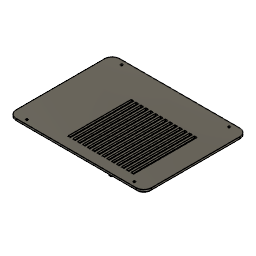
Mini PC Lid V2 (Autodesk Fusion 360 design; units mm, degrees)
Autodesk Fusion 360 part; units mm, degrees
sketch "Sketch1" plane through (0, 0, 0) normal (0, 0, 1) x (1, 0, 0)
  line L0 (10, 0) -> (200, 0)
  line L1 (210, 10) -> (210, 150)
  line L2 (200, 160) -> (10, 160)
  line L3 (0, 150) -> (0, 10)
  arc A0 (10, 160) -> (0, 150) centre (10, 150) ccw
  arc A1 (210, 150) -> (200, 160) centre (200, 150) ccw
  arc A2 (200, 0) -> (210, 10) centre (200, 10) ccw
  arc A3 (0, 10) -> (10, 0) centre (10, 10) ccw
  line L4 (200, 162) -> (10, 162)
  arc A4 (10, 162) -> (-2, 150) centre (10, 150) ccw
  line L5 (-2, 150) -> (-2, 10)
  arc A5 (-2, 10) -> (10, -2) centre (10, 10) ccw
  line L6 (10, -2) -> (200, -2)
  arc A6 (200, -2) -> (212, 10) centre (200, 10) ccw
  line L7 (212, 10) -> (212, 150)
  arc A7 (212, 150) -> (200, 162) centre (200, 150) ccw
  line L8 (200, 155) -> (10, 155)
  arc A8 (10, 155) -> (5, 150) centre (10, 150) ccw
  line L9 (5, 150) -> (5, 10)
  arc A9 (5, 10) -> (10, 5) centre (10, 10) ccw
  line L10 (10, 5) -> (200, 5)
  arc A10 (200, 5) -> (205, 10) centre (200, 10) ccw
  line L11 (205, 10) -> (205, 150)
  arc A11 (205, 150) -> (200, 155) centre (200, 150) ccw
  circle A12 centre (20, 5) radius 1.1
  circle A13 centre (20, 5) radius 3
  circle A14 centre (66, 85) radius 1.1
  circle A15 centre (186, 76) radius 1.1
  circle A16 centre (150, 9) radius 1.1
  circle A17 centre (150, 9) radius 3
  circle A18 centre (66, 85) radius 3
  circle A19 centre (186, 76) radius 3
  line L12 (105, 162) -> (105, -2) construction
  line L13 (212, 80) -> (-2, 80) construction
  circle A20 centre (190, 5) radius 3
  circle A21 centre (190, 5) radius 1.1
  circle A22 centre (20, 155) radius 3
  circle A23 centre (20, 155) radius 1.1
  circle A24 centre (190, 155) radius 3
  circle A25 centre (190, 155) radius 1.1
  point P0 (210, 0)
  point P1 (0, 160)
  dimension "d1" = 210
  dimension "d2" = 160
  dimension "d4" = 10
  dimension "d5" = 2
  dimension "d6" = -5
  dimension "d9" = 2.2
  dimension "d10" = 6
  dimension "d11" = 20
  dimension "d12" = 5
  dimension "d13" = 2.2
  dimension "d14" = 2.2
  dimension "d15" = 2.2
  dimension "d17" = 75
  dimension "d18" = 84
  dimension "d19" = 24
  dimension "d21" = 60
  dimension "d22" = 9
  dimension "d23" = 66
  dimension "d24" = 6
  dimension "d25" = 6
  dimension "d26" = 6
  dimension "d31" = 170
  dimension "d32" = 150
  constraint horizontal L0
  constraint vertical L1
  constraint horizontal L2
  constraint vertical L3
  constraint coincident P1 L2
  constraint coincident P1 L3
  constraint tangent L2 A0
  constraint tangent L3 A0
  constraint tangent L1 A1
  constraint tangent L2 A1
  constraint equal A0 A1
  constraint coincident P0 L0
  constraint coincident P0 L1
  constraint tangent L0 A2
  constraint tangent L1 A2
  constraint equal A0 A2
  constraint coincident origin L0
  constraint coincident origin L3
  constraint tangent L0 A3
  constraint tangent L3 A3
  constraint equal A0 A3
  constraint concentric A12 A13
  constraint concentric A16 A17
  constraint concentric A14 A18
  constraint concentric A15 A19
  constraint midpoint L4 L12.start
  constraint midpoint L6 L12.end
  constraint midpoint L7 L13.start
  constraint midpoint L5 L13.end
  measures "d1" distance of origin P0
  measures "d2" distance of origin P1
  measures "d4" radius of A0
  measures "d9" diameter of A12
  measures "d10" diameter of A13
  measures "d11" distance of L3 A12.centre
  measures "d12" distance of L0 A12.centre
  measures "d13" diameter of A14
  measures "d14" diameter of A15
  measures "d15" diameter of A16
  measures "d17" distance of L2 A14.centre
  measures "d18" distance of L2 A15.centre
  measures "d19" distance of L1 A15.centre
  measures "d21" distance of L1 A16.centre
  measures "d22" distance of L0 A16.centre
  measures "d23" distance of L3 A14.centre
  measures "d24" diameter of A17
  measures "d25" diameter of A18
  measures "d26" diameter of A19
extrude "Extrude1" add sketch "Sketch1" against normal blind 1 contours L0 L1 L2 L3 A0 A1 A2 A3 | L4 A4 L5 A5 L6 A6 L7 A7 | L8 A8 L9 A9 L10 A10 L11 A11 A13 A20 A22 A24 | L8 A24 A25 | L8 A24 A25 | L8 A25 | L8 A25 | L8 A22 A23 | L8 A22 A23 | L8 A23 | L8 A23 | L10 A20 A21 | L10 A20 A21 | L10 A21 | L10 A21 | L10 A12 A13 | L10 A12 A13 | L10 A12 | L10 A12 | A14 | A15 | A16 | A17 | A18 | A19
extrude "Extrude2" add sketch "Sketch1" against normal blind 3 contours L0 L1 L2 L3 A0 A1 A2 A3 | L8 A24 A25 | L8 A24 A25 | L8 A22 A23 | L8 A22 A23 | L10 A20 A21 | L10 A20 A21 | L10 A12 A13 | L10 A12 A13 | A17 | A18 | A19
sketch "Sketch3" plane through (0, 0, -1) normal (0, 0, -1) x (1, 0, 0)
  arc A0 (200, -162) -> (212, -150) centre (200, -150) ccw
  line L0 (212, -150) -> (212, -10)
  arc A1 (212, -10) -> (200, 2) centre (200, -10) ccw
  line L1 (200, 2) -> (10, 2)
  arc A2 (10, 2) -> (-2, -10) centre (10, -10) ccw
  line L2 (-2, -10) -> (-2, -150)
  arc A3 (-2, -150) -> (10, -162) centre (10, -150) ccw
  line L3 (10, -162) -> (200, -162)
  circle A4 centre (190, -155) radius 2.25
  circle A5 centre (20, -155) radius 2.25
  circle A6 centre (66, -85) radius 2.25
  circle A7 centre (186, -76) radius 2.25
  circle A8 centre (190, -5) radius 2.25
  circle A9 centre (150, -9) radius 2.25
  circle A10 centre (20, -5) radius 2.25
  line L4 (10, 0) -> (200, 0)
  arc A11 (210, -10) -> (200, 0) centre (200, -10) ccw
  line L5 (210, -10) -> (210, -150)
  arc A12 (200, -160) -> (210, -150) centre (200, -150) ccw
  line L6 (200, -160) -> (10, -160)
  arc A13 (0, -150) -> (10, -160) centre (10, -150) ccw
  line L7 (0, -150) -> (0, -10)
  arc A14 (10, 0) -> (0, -10) centre (10, -10) ccw
  dimension "d38" = 4.5
  dimension "d39" = 4.5
  dimension "d40" = 4.5
  dimension "d41" = 4.5
  dimension "d42" = 4.5
  dimension "d43" = 4.5
  dimension "d44" = 4.5
  measures "d38" diameter of A4
  measures "d39" diameter of A5
  measures "d40" diameter of A6
  measures "d41" diameter of A7
  measures "d42" diameter of A8
  measures "d43" diameter of A9
  measures "d44" diameter of A10
extrude "Extrude5" cut 4 faces at (189.4633, 4.7506, -1) (20.2286, 5.396, -1) (20.2286, 154.7133, -1) (189.8112, 154.6587, -1) along direction (0, 0, -1) up to surface end surface through (0, 0, 0) normal (0, 0, 1) offset 0
chamfer "Chamfer1" distance 0.5 angle 45 4 edges at (188.9744, 155.3978, 0) (188.9744, 5.3978, 0) (18.9744, 5.3978, 0) (18.9744, 155.3978, 0)
extrude "Extrude6" add 3 faces at (184.3747, 74.2886, -3) (152.3555, 8.851, -3) (64.3747, 83.2886, -3) along direction (0, 0, -1) blind 8
chamfer "Chamfer2" distance 2 angle 45 3 edges at (183.203, 74.9152, -1) (147.203, 7.9152, -1) (63.203, 83.9152, -1)
sketch "Sketch4" plane through (0, 0, -1) normal (0, 0, -1) x (1, 0, 0)
  circle A0 centre (186, -76) radius 5
  arc A1 (147, -5) -> (153, -5) centre (150, -9) ccw
  line L0 (147, -5) -> (23, -5)
  arc A2 (17, -5) -> (23, -5) centre (20, -5) ccw
  line L1 (17, -5) -> (10, -5)
  arc A3 (10, -5) -> (5, -10) centre (10, -10) ccw
  line L2 (5, -10) -> (5, -150)
  arc A4 (5, -150) -> (10, -155) centre (10, -150) ccw
  line L3 (10, -155) -> (17, -155)
  arc A5 (23, -155) -> (17, -155) centre (20, -155) ccw
  line L4 (23, -155) -> (187, -155)
  arc A6 (193, -155) -> (187, -155) centre (190, -155) ccw
  line L5 (193, -155) -> (200, -155)
  arc A7 (200, -155) -> (205, -150) centre (200, -150) ccw
  line L6 (205, -150) -> (205, -10)
  arc A8 (205, -10) -> (200, -5) centre (200, -10) ccw
  line L7 (200, -5) -> (193, -5)
  arc A9 (187, -5) -> (193, -5) centre (190, -5) ccw
  line L8 (187, -5) -> (153, -5)
  circle A10 centre (66, -85) radius 5
  line L9 (75, -115) -> (79, -115)
  line L10 (79, -115) -> (79, -15)
  line L11 (79, -15) -> (75, -15)
  line L12 (75, -15) -> (75, -115)
  line L13 (82.6923, -15) -> (82.6923, -115)
  line L14 (82.6923, -115) -> (86.6923, -115)
  line L15 (86.6923, -115) -> (86.6923, -15)
  line L16 (86.6923, -15) -> (82.6923, -15)
  line L17 (90.3846, -15) -> (90.3846, -115)
  line L18 (90.3846, -115) -> (94.3846, -115)
  line L19 (94.3846, -115) -> (94.3846, -15)
  line L20 (94.3846, -15) -> (90.3846, -15)
  line L21 (98.0769, -15) -> (98.0769, -115)
  line L22 (98.0769, -115) -> (102.0769, -115)
  line L23 (102.0769, -115) -> (102.0769, -15)
  line L24 (102.0769, -15) -> (98.0769, -15)
  line L25 (105.7692, -15) -> (105.7692, -115)
  line L26 (105.7692, -115) -> (109.7692, -115)
  line L27 (109.7692, -115) -> (109.7692, -15)
  line L28 (109.7692, -15) -> (105.7692, -15)
  line L29 (113.4615, -15) -> (113.4615, -115)
  line L30 (113.4615, -115) -> (117.4615, -115)
  line L31 (117.4615, -115) -> (117.4615, -15)
  line L32 (117.4615, -15) -> (113.4615, -15)
  line L33 (121.1538, -15) -> (121.1538, -115)
  line L34 (121.1538, -115) -> (125.1538, -115)
  line L35 (125.1538, -115) -> (125.1538, -15)
  line L36 (125.1538, -15) -> (121.1538, -15)
  line L37 (128.8462, -15) -> (128.8462, -115)
  line L38 (128.8462, -115) -> (132.8462, -115)
  line L39 (132.8462, -115) -> (132.8462, -15)
  line L40 (132.8462, -15) -> (128.8462, -15)
  line L41 (136.5385, -15) -> (136.5385, -115)
  line L42 (136.5385, -115) -> (140.5385, -115)
  line L43 (140.5385, -115) -> (140.5385, -15)
  line L44 (140.5385, -15) -> (136.5385, -15)
  line L45 (144.2308, -15) -> (144.2308, -115)
  line L46 (144.2308, -115) -> (148.2308, -115)
  line L47 (148.2308, -115) -> (148.2308, -15)
  line L48 (148.2308, -15) -> (144.2308, -15)
  line L49 (151.9231, -15) -> (151.9231, -115)
  line L50 (151.9231, -115) -> (155.9231, -115)
  line L51 (155.9231, -115) -> (155.9231, -15)
  line L52 (155.9231, -15) -> (151.9231, -15)
  line L53 (159.6154, -15) -> (159.6154, -115)
  line L54 (159.6154, -115) -> (163.6154, -115)
  line L55 (163.6154, -115) -> (163.6154, -15)
  line L56 (163.6154, -15) -> (159.6154, -15)
  line L57 (167.3077, -15) -> (167.3077, -115)
  line L58 (167.3077, -115) -> (171.3077, -115)
  line L59 (171.3077, -115) -> (171.3077, -15)
  line L60 (171.3077, -15) -> (167.3077, -15)
  line L61 (175, -15) -> (175, -115)
  line L62 (175, -115) -> (179, -115)
  line L63 (179, -115) -> (179, -15)
  line L64 (179, -15) -> (175, -15)
  dimension "d53" = 4
  dimension "d54" = 100
  dimension "d57" = 100
  dimension "d58" = 0
  constraint horizontal L9
  constraint vertical L10
  constraint horizontal L11
  constraint vertical L12
  measures "d53" distance of L9.start L9.end
  measures "d54" distance of L9.start L11.end
extrude "Extrude7" cut sketch "Sketch4" against normal blind 2 contours L9 L10 L11 L12 | L13 L14 L15 L16 | L17 L18 L19 L20 | L21 L22 L23 L24 | L25 L26 L27 L28 | L29 L30 L31 L32 | L33 L34 L35 L36 | L37 L38 L39 L40 | L41 L42 L43 L44 | L45 L46 L47 L48 | L49 L50 L51 L52 | L53 L54 L55 L56 | L57 L58 L59 L60 | L61 L62 L63 L64
extrude "Extrude8" add 1 faces at (23.6667, 91.6667, 0) along direction (0, 0, 1) blind 2
equation "BoxRadius = 10 mm"
equation "d4 = BoxRadius"
equation "HolesRadius = 2.2 mm"
equation "HolesOuterRadius = 6 mm"
equation "d9 = HolesRadius"
equation "d10 = HolesOuterRadius"
equation "d13 = HolesRadius"
equation "d14 = HolesRadius"
equation "d15 = HolesRadius"
equation "d24 = HolesOuterRadius"
equation "d25 = HolesOuterRadius"
equation "d26 = HolesOuterRadius"
equation "BoltHead = 4.5 mm"
equation "d38 = BoltHead"
equation "d39 = BoltHead"
equation "d40 = BoltHead"
equation "d41 = BoltHead"
equation "d42 = BoltHead"
equation "d43 = BoltHead"
equation "d44 = BoltHead"
